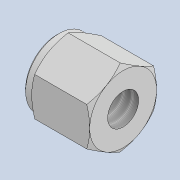
# Autodesk Inventor part: Nut for Precision Compression Fitting
Saved by Autodesk Inventor 2022.5 (Build 265521000, 521)
## iProperties
Created: 2023-08-31
Part Number: Nut for Precision Compression Fitting
Material: Generic
Document SubType Name: Modeling
Designer: SB13FLLT004
Density: 1 g/cm^3
Appearance: Default
Author: Shannon Toole
Autodesk Inventor part; units mm, degrees
ref_plane "YZ Plane" through (0, 0, 0) normal (1, 0, 0) x (0, 1, 0)
sketch "Sketch1: Hex" plane through (0, 0, 0) normal (1, 0, 0) x (0, 1, 0)
  line L0 (-2.2914, 3.9688) -> (2.2914, 3.9687)
  line L1 (2.2914, 3.9687) -> (4.5827, 0)
  line L2 (4.5827, 0) -> (2.2914, -3.9688)
  line L3 (2.2914, -3.9688) -> (-2.2914, -3.9688)
  line L4 (-2.2914, -3.9688) -> (-4.5827, 0)
  line L5 (-4.5827, 0) -> (-2.2914, 3.9688)
  circle A0 centre (0, 0) radius 0.87
  point P0 (0, 3.9687)
  point P1 (0, -3.9688)
  dimension "hex_angle" = 120
  dimension "hex_size" = 7.9375
  dimension "d1" = 1.7399
  constraints: 12 end point, 3 parallel, 3 vertical alignment, 2 equal length, 2 horizontal alignment, 2 midpoint, 1 centre point, 1 coincident
  measures "hex_angle" angle of L1 L0
  measures "hex_size" distance between parallel lines of L3 L0
  measures "d1" diameter of A0
extrude "Ex: Hex" add sketch "Sketch1: Hex" against normal blind 6.8898 contours L0 L1 L2 L3 L4 L5 | A0
hole "Hole: Tap" [suppressed]
hole "Hole: Thread" at (0, 0, 0) direction (-1, 0, 0) diameter 3.683 depth 5.842 thread size "10-24 UNC" class "2B" standard "ANSI Unified Screw Threads"
sketch "Sketch2: Top" plane through (-6.8898, 0, 0) normal (1, 0, 0) x (0, 1, 0)
  circle A0 centre (0, 0) radius 3.9687
  circle A1 centre (0, 0) radius 3.7147
  dimension "d4" = 7.9375
  dimension "d5" = 7.4295
  constraints: 2 centre point, 2 coincident
  measures "d4" diameter of A0
  measures "d5" diameter of A1
extrude "Ex: Top" add sketch "Sketch2: Top" against normal blind 0.9843 contours A0 | A1
hole "Hole: Tubing" at (0, 0, 0) direction (-1, 0, 0) diameter 1.7399 end through all
chamfer "Chamfer1: Top (side)" distance 0.254 angle 45 1 edges at (-7.874, -3.9687, 0)
chamfer "Chamfer2: Top (hole)" distance 0.254 angle 45 1 edges at (-7.874, 0, 0.87)
sketch "Sketch3: Reference: Nut Chamfer" plane through (0, 0, 0) normal (1, 0, 0) x (0, 0, -1)
  circle A0 centre (0, 0) radius 3.9688
  line L0 (3.9688, 2.2914) -> (0, 4.5827) projected
  constraints: 1 centre point, 1 coincident, 1 tangent
ref_plane "Work Plane1" through (0, 2.2914, -3.9688) normal (0, 0.8660254, 0.5) x (-1, 0, 0)
sketch "Sketch4: Chamfer (nut)" plane through (0, 0, 0) normal (0, 0.8660254, 0.5) x (-1, 0, 0)
  line L0 (0, -3.9688) -> (0, -4.5827)
  line L1 (0, -4.5827) -> (0.3545, -4.5827)
  line L2 (0.3545, -4.5827) -> (0, -3.9688)
  line L3 (0, 3.9688) -> (0, -3.9688) projected
  line L4 (8.2677, 0) -> (-1.378, 0) projected
  line L5 (0, -4.5827) -> (6.8898, -4.5827) projected
  point P0 (0, 0)
  dimension "chamfer_angle" = 30
  constraints: 6 end point, 1 collinear, 1 vertical
  measures "chamfer_angle" angle of L2 L0
revolve "Revolution: Chamfer (nut)" cut sketch "Sketch4: Chamfer (nut)" angle 360 about axis through (-10, 0, 0) along (1, 0, 0)
ref_plane "Work Plane2: Hex Center" through (-3.4449, 0, 0) normal (1, 0, 0) x (0, 0, -1)
mirror "Mirror: Chamfer (nut)" about plane through (-3.4449, 0, 0) normal (1, 0, 0) of "Revolution: Chamfer (nut)"
body "Solid1"
